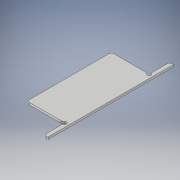
# Autodesk Inventor part: Maze Wall Alignment Jig
Saved by Autodesk Inventor 2019 (Build 230136000, 136)
## iProperties
Created: 2019-02-13
Part Number: Maze Wall Alignment Jig
Material: Generic
Document SubType Name: Modeling
Designer: Billy
Density: 1 g/cm^3
Appearance: Default
Author: Billy
Autodesk Inventor part; units mm, degrees
ref_plane "YZ Plane" through (0, 0, 0) normal (1, 0, 0) x (0, 1, 0)
ref_plane "XZ Plane" through (0, 0, 0) normal (0, 1, 0) x (-1, 0, 0)
ref_plane "XY Plane" through (0, 0, 0) normal (0, 0, 1) x (1, 0, 0)
sketch "Sketch1" plane through (0, 0, 0) normal (0, 1, 0) x (-1, 0, 0)
  line L0 (55, -30) -> (55, -135.5)
  line L1 (0, -165.5) -> (0, 0)
  line L2 (52, -27) -> (9.6098, -27)
  line L3 (0, -27) -> (0, 0)
  line L4 (52, -138.5) -> (9.6098, -138.5)
  line L5 (0, -138.5) -> (0, -165.5)
  line L6 (0, 0) -> (2, 0)
  line L7 (5, -3) -> (5, -22.3902)
  line L8 (0, -27) -> (0, 0)
  line L9 (0, -165.5) -> (2, -165.5)
  line L10 (5, -162.5) -> (5, -143.1098)
  line L11 (0, -138.5) -> (0, -165.5)
  arc A0 (3.6364, -24.9046) -> (7.0954, -28.3636) centre (5, -27) ccw
  arc A1 (7.0954, -137.1364) -> (3.6364, -140.5954) centre (5, -138.5) ccw
  arc A2 (55, -30) -> (52, -27) centre (52, -30) ccw
  arc A3 (52, -138.5) -> (55, -135.5) centre (52, -135.5) ccw
  arc A4 (9.6098, -27) -> (7.0954, -28.3636) centre (9.6098, -30) ccw
  arc A5 (3.6364, -24.9046) -> (5, -22.3902) centre (2, -22.3902) ccw
  arc A6 (7.0954, -137.1364) -> (9.6098, -138.5) centre (9.6098, -135.5) ccw
  arc A7 (5, -143.1098) -> (3.6364, -140.5954) centre (2, -143.1098) ccw
  arc A8 (5, -3) -> (2, 0) centre (2, -3) ccw
  arc A9 (2, -165.5) -> (5, -162.5) centre (2, -162.5) ccw
  point P0 (5, -24.5)
  point P1 (5, -141)
  point P2 (7.5, -27)
  point P3 (7.5, -138.5)
  dimension "d8" = 3
  dimension "d9" = 3
  constraints: 24 end point, 24 point on circle, 16 tangent, 10 centre point, 6 equal radius, 4 point on line, 3 parallel, 2 horizontal, 2 perpendicular
  measures "d8" radius of A2
  measures "d9" radius of A8
extrude "Extrusion1" add sketch "Sketch1" along normal blind 3
body "Solid1"
